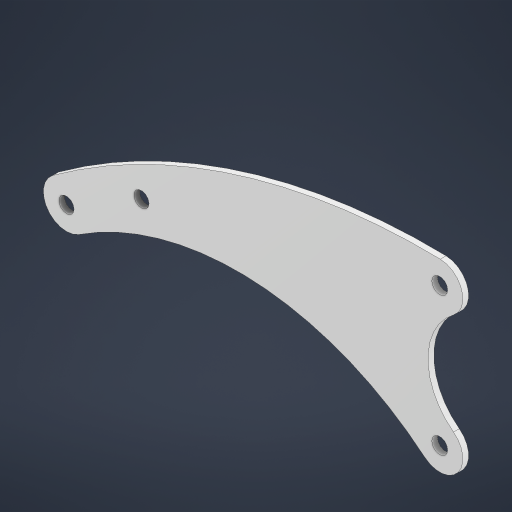
# Autodesk Inventor part: triball_jig
Saved by Autodesk Inventor 2024 (Build 280153000, 153)
## iProperties
Created: 2023-11-21
Part Number: triball_jig
Material: Acetal Resin, White
Document SubType Name: Sheet Metal
Designer: avere
Density: 1.425 g/cm^3
Appearance: Smooth - White
Flat Pattern Width: 5.07905 cm
Flat Pattern Length: 11.5437 cm
Flat Pattern Area: 58.631 cm^2
Sheet Metal Rule: Default_mm
Sheet Metal Width: 2.000 in
Sheet Metal Length: 4.545 in
Sheet Metal Area: 9.088 in^2
Author: avere
Autodesk Inventor part; units mm, degrees
ref_plane "YZ Plane" through (0, 0, 0) normal (1, 0, 0) x (0, 1, 0)
ref_plane "XZ Plane" through (0, 0, 0) normal (0, 1, 0) x (-1, 0, 0)
ref_plane "XY Plane" through (0, 0, 0) normal (0, 0, 1) x (1, 0, 0)
sketch "Block1" plane through (0, 0, 0) normal (0, 0, 1) x (1, 0, 0)
  circle A0 centre (47.0944, 34.7657) radius 2.1844
  circle A1 centre (-55.5339, 40.771) radius 2.0955
  arc A2 (-59.2675, 45.9074) -> (-52.0623, 35.454) centre (-55.5339, 40.771) ccw
  arc A3 (43.0264, 29.8899) -> (53.4444, 34.7657) centre (47.0944, 34.7657) ccw
  arc A4 (43.0264, 29.8899) -> (-52.0623, 35.454) centre (-8.279, -31.6038) ccw
  circle A5 centre (47.0944, 72.8657) radius 2.1844
  arc A6 (53.4444, 72.8657) -> (47.2364, 79.2141) centre (47.0944, 72.8657) ccw
  arc A7 (47.2364, 79.2141) -> (-59.2675, 45.9074) centre (43.3348, -95.2454) ccw
  circle A8 centre (-34.925, 52.3875) radius 2.0955
  point P0 (37.587, 35.3505)
  dimension "d2" = 12.7
  dimension "d3" = 12.7
  dimension "d4" = 12.7
  dimension "d9" = 4.191
  measures "d2" diameter of A2
  measures "d3" diameter of A3
  measures "d4" diameter of A6
  measures "d9" diameter of A8
sketch "Sketch1" plane through (0, 0, 0) normal (0, 0, 1) x (1, 0, 0)
  arc A0 (3.787, 33.0028) -> (0.142, 44.4484) centre (0, 38.1) ccw
  arc A1 (-4.068, -4.8758) -> (3.787, 5.0972) centre (0, 0) ccw
  arc A2 (3.787, 33.0028) -> (3.787, 5.0972) centre (14.1532, 19.05) ccw
  circle A3 centre (0, 0) radius 2.1844
  circle A4 centre (-102.6283, 6.0053) radius 2.0955
  arc A5 (-106.3619, 11.1417) -> (-99.1567, 0.6883) centre (-102.6283, 6.0053) ccw
  arc A6 (-4.068, -4.8758) -> (6.35, 0) centre (0, 0) ccw
  arc A7 (-4.068, -4.8758) -> (-99.1567, 0.6883) centre (-55.3735, -66.3695) ccw
  circle A8 centre (0, 38.1) radius 2.1844
  arc A9 (6.35, 38.1) -> (0.142, 44.4484) centre (0, 38.1) ccw
  arc A10 (0.142, 44.4484) -> (-106.3619, 11.1417) centre (-3.7596, -130.0112) ccw
  circle A11 centre (-82.0194, 17.6218) radius 2.0955
  point P0 (6.35, 0)
  point P1 (6.35, 38.1)
  constraints: 6 point on circle, 3 centre point, 2 tangent, 6 other
extrude "Extrusion1" add sketch "Sketch1" along normal blind 1.5875
equation "\"BendRadius\" = Thickness"
equation "\"BendReliefWidth\" = Thickness"
equation "\"BendReliefDepth\" = 0.5 * Thickness"
equation "\"CornerReliefSize\" = 4 * Thickness"
equation "\"MinimumRemnant\" = 2 * Thickness"
equation "\"TransitionRadius\" = BendRadius"
equation "\"JacobiRadiusSize\" = BendRadius"
equation "\"GapSize\" = Thickness"
equation "\"Thickness\" = 1.5875"
body "Solid1"
